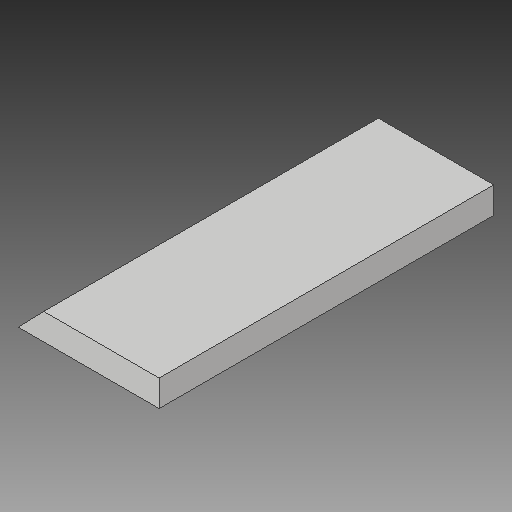
# Autodesk Inventor part: slant_front
Saved by Autodesk Inventor 2017 (Build 210142000, 142)
## iProperties
Created: 2019-03-22
Part Number: slant_front
Material: Generic
Document SubType Name: Modeling
Designer: Mitch
Density: 1 g/cm^3
Appearance: Default
Mass: 424.751 g
Surface Area: 591.007 cm^2
Volume: 424.751 cm^3
Author: Mitch
Autodesk Inventor part; units mm, degrees
ref_plane "YZ Plane" through (0, 0, 0) normal (1, 0, 0) x (0, 1, 0)
ref_plane "XZ Plane" through (0, 0, 0) normal (0, 1, 0) x (-1, 0, 0)
ref_plane "XY Plane" through (0, 0, 0) normal (0, 0, 1) x (1, 0, 0)
sketch "Sketch1" plane through (0, 0, 0) normal (0, 1, 0) x (-1, 0, 0)
  line L0 (0, 0) -> (101.6, 0)
  line L1 (101.6, 0) -> (101.6, -241.3)
  line L2 (101.6, -241.3) -> (0, -241.3)
  line L3 (0, -241.3) -> (0, 0)
  dimension "d0" = 101.6
  dimension "d1" = 241.3
  constraints: 8 end point, 2 parallel, 1 horizontal, 1 perpendicular
  measures "d0" distance of L1.end L2.end
  measures "d1" distance of L0.end L1.end
extrude "Extrusion1" add sketch "Sketch1" along normal blind 19.05
sketch "Sketch2" plane through (-101.6, 0, 0) normal (0, 0, 1) x (1, 0, 0)
  line L0 (0, 0) -> (18.3964, 19.05)
  line L1 (0, 0) -> (0, 19.05)
  line L2 (0, 19.05) -> (18.3964, 19.05)
  line L3 (0, 19.05) -> (101.6, 19.05) projected
  constraints: 6 end point, 1 collinear, 1 vertical
extrude "Extrusion2" cut sketch "Sketch2" against normal blind 254
body "Solid1"
